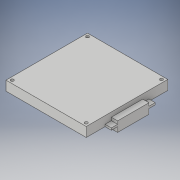
# Autodesk Inventor part: Keypad
Saved by Autodesk Inventor 2019 (Build 230136000, 136)
## iProperties
Created: 2019-03-10
Part Number: Keypad
Material: Generic
Document SubType Name: Modeling
Designer: savo
Density: 1 g/cm^3
Appearance: Default
Author: savo
Autodesk Inventor part; units mm, degrees
ref_plane "YZ Plane" through (0, 0, 0) normal (1, 0, 0) x (0, 1, 0)
ref_plane "XZ Plane" through (0, 0, 0) normal (0, 1, 0) x (-1, 0, 0)
ref_plane "XY Plane" through (0, 0, 0) normal (0, 0, 1) x (1, 0, 0)
sketch "Sketch1" plane through (0, 0, 0) normal (0, 1, 0) x (-1, 0, 0)
  line L0 (0, 0) -> (64, 0)
  line L1 (64, 0) -> (64, -65)
  line L2 (64, -65) -> (0, -65)
  line L3 (0, -65) -> (0, 0)
  line L4 (0, -15) -> (-5, -15)
  line L5 (-5, -15) -> (-5, -50)
  line L6 (-5, -50) -> (0, -50)
  line L7 (0, -50) -> (0, -15)
  dimension "d0" = 64
  dimension "d1" = 65
  dimension "d2" = 5
  dimension "d3" = 15
  dimension "d4" = 15
  constraints: 16 end point, 4 parallel, 2 horizontal, 2 perpendicular, 1 point on line
  measures "d0" distance of L1.end L2.end
  measures "d1" distance of L0.end L1.end
  measures "d2" distance of L5.end L6.end
  measures "d3" distance between parallel lines of L0 L4
  measures "d4" distance between parallel lines of L2 L6
extrude "Extrusion1" add sketch "Sketch1" along normal blind 1.6
sketch "Sketch2" plane through (0, 0, 0) normal (0, -1, 0) x (1, 0, 0)
  line L0 (5, -15) -> (5, -50) projected
  line L1 (5, -20) -> (0, -20)
  line L2 (0, -20) -> (0, -45)
  line L3 (0, -45) -> (5, -45)
  line L4 (5, -45) -> (5, -20)
  point P0 (0, 0)
  point P1 (5, -32.5)
  dimension "d7" = 5
  dimension "d8" = 25
  constraints: 8 end point, 2 midpoint, 2 parallel, 1 horizontal, 1 perpendicular, 1 point on line
  measures "d7" distance of L3.end L2.end
  measures "d8" distance of L2.end L1.end
extrude "Extrusion2" add sketch "Sketch2" along normal mid plane 8
sketch "Sketch3" plane through (0, 1.6, 0) normal (0, 1, 0) x (1, 0, 0)
  line L0 (0, 0) -> (0, 15) projected
  line L1 (-64, 65) -> (-64, 0) projected
  line L2 (0, 0) -> (-64, 0)
  line L3 (-64, 0) -> (-64, 65)
  line L4 (-64, 65) -> (0, 65)
  line L5 (0, 65) -> (0, 0)
  constraints: 8 end point, 2 parallel, 1 horizontal, 1 perpendicular
extrude "Extrusion3" add sketch "Sketch3" along normal blind 6
sketch "Sketch4" plane through (0, 7.6, 0) normal (0, 1, 0) x (1, 0, 0)
  line L0 (-64, 0) -> (0, 0) projected
  line L1 (-64, 65) -> (-64, 0) projected
  point P0 (-61.5, 2.5)
  point P1 (-2.5, 2.5)
  point P2 (-61.5, 62.5)
  point P3 (-2.5, 62.5)
  dimension "d13" = 2.5
  dimension "d14" = 2.5
  dimension "d17" = 59
  dimension "d20" = 60
  constraints: 1 horizontal, 1 vertical, 3 other
  measures "d13" distance from line of L0 point (-61.5, 2.5)
  measures "d14" distance from line of point (-61.5, 2.5) L1
  measures "d17" distance of point (-61.5, 2.5) point (-2.5, 2.5)
  measures "d20" distance of point (-61.5, 2.5) point (-61.5, 62.5)
hole "Hole1" at (-61.5, 7.6, -2.5) at (-2.5, 7.6, -2.5) at (-61.5, 7.6, -62.5) at (-2.5, 7.6, -62.5) direction (0, -1, 0) diameter 2.4 end through all clearance for "Flat Head Machine Screw" size "M2" standard "Ansi Metric M Profile"
body "Solid1"
